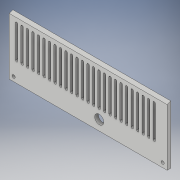
# Autodesk Inventor part: Gehaeuse_IN12_Rueckwand
Saved by Autodesk Inventor 2019 (Build 230136000, 136)
## iProperties
Created: 2019-11-29
Part Number: Gehaeuse_IN12_Rueckwand
Material: Generisch
Document SubType Name: Modeling
Designer: grubi
Density: 1 g/cm^3
Appearance: Vorgabe
Author: grubi
Autodesk Inventor part; units mm, degrees
ref_plane "YZ Plane" through (0, 0, 0) normal (1, 0, 0) x (0, 1, 0)
ref_plane "XZ Plane" through (0, 0, 0) normal (0, 1, 0) x (-1, 0, 0)
ref_plane "XY Plane" through (0, 0, 0) normal (0, 0, 1) x (1, 0, 0)
sketch "Skizze1" plane through (0, 0, 0) normal (0, 0, 1) x (1, 0, 0)
  line L0 (-86.1, -31) -> (86.1, -31)
  line L1 (86.1, -31) -> (86.1, 31)
  line L2 (86.1, 31) -> (-86.1, 31)
  line L3 (-86.1, 31) -> (-86.1, -31)
  line L4 (-86.1, -31) -> (86.1, 31) construction
  line L5 (86.1, -31) -> (-86.1, 31) construction
  point P0 (0, 0)
  dimension "d0" = 62
  dimension "d1" = 172.2
  constraints: 12 end point, 2 midpoint, 2 parallel, 1 horizontal, 1 perpendicular
  measures "d0" distance of L2.end L0.start
  measures "d1" distance of L0.start L0.end
extrude "Extrusion1" add sketch "Skizze1" along normal blind 4
sketch "Skizze2" plane through (86.1, -31, 0) normal (1, 0, 0) x (0, 0, -1)
  line L0 (0, 62) -> (-4, 62) projected
  line L1 (-4, 62) -> (0, 63.4559)
  line L2 (0, 63.4559) -> (0, 62)
  point P0 (0, 31)
  dimension "d4" = 20
  constraints: 4 end point, 1 perpendicular
  measures "d4" angle of L1 L0
extrude "Extrusion2" add sketch "Skizze2" against normal up to surface (172.2 mm away)
sketch "Skizze3" plane through (0, 0, 4) normal (0, 0, 1) x (1, 0, 0)
  line L0 (86.1, -31) -> (86.1, 31) projected
  line L1 (-86.1, -31) -> (86.1, -31) projected
  point P0 (0, 0)
  point P1 (12.1, -20)
  dimension "d7" = 74
  dimension "d8" = 11
  measures "d7" distance from line of point (12.1, -20) L0
  measures "d8" distance from line of L1 point (12.1, -20)
hole "Bohrung1" at (12.1, -20, 4) direction (0, 0, -1) diameter 10 depth 15 tip angle 118
sketch "Skizze4" plane through (0, 0, 4) normal (0, 0, 1) x (1, 0, 0)
  line L0 (0, 0) -> (0, 31.3985) construction
  line L1 (-86.1, -31) -> (86.1, -31) projected
  point P0 (-81.203, -26.1)
  point P1 (81.203, -26.1)
  dimension "d16" = 162.406
  dimension "d17" = 4.9
  constraints: 2 end point, 1 symmetric about line, 1 vertical
  measures "d16" distance of point (81.203, -26.1) point (-81.203, -26.1)
  measures "d17" distance from line of point (-81.203, -26.1) L1
hole "Bohrung2" at (-81.203, -26.1, 4) at (81.203, -26.1, 4) direction (0, 0, -1) diameter 3.4 depth 15 tip angle 118 clearance for "Flachkopfsenkschraube DIN EN ISO 2009" size "M3" standard "DIN"
sketch "Skizze5" plane through (0, 0, 4) normal (0, 0, 1) x (1, 0, 0)
  line L0 (0, -9.5) -> (0, 25.5) construction
  line L1 (-1.3061, -9.5) -> (-1.3061, 25.5)
  line L2 (1.3061, 25.5) -> (1.3061, -9.5)
  arc A0 (-1.3061, -9.5) -> (1.3061, -9.5) centre (0, -9.5) ccw
  arc A1 (1.3061, 25.5) -> (-1.3061, 25.5) centre (0, 25.5) ccw
  point P0 (0, 0)
  point P1 (0, 8)
  dimension "d25" = 35
  dimension "d26" = 8
  constraints: 8 end point, 4 point on circle, 4 tangent, 2 centre point, 1 midpoint, 1 parallel, 1 vertical
  measures "d25" distance of L0.start L0.end
  measures "d26" distance of point (0, 0) point (0, 8)
extrude "Extrusion3" cut sketch "Skizze5" against normal through all
pattern_linear "Rechteckige Anordnung1" count 26 spacing 6 along (-1, 0, 0) of "Extrusion3" first direction both ways yes
